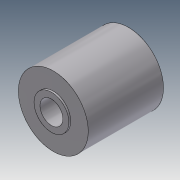
# Autodesk Inventor part: J008110
Saved by Autodesk Inventor 2018.3 (Build 223284000, 284)
## iProperties
Created: 2018-10-11
Material: ALUMINUM, 6061-T651
Vendor: HHMI: JRC - ID&F
Document SubType Name: Modeling
Designer: arnoldj
Density: 2.7 g/cm^3
Appearance: Metal-AL-6061 (Machined)
Part Number: J008110
Description: VP SPACER LOWER CYL
Project: COMMON
RuleStatus: InUse
AfterDocSave0: file://Part Number Cleaner
LAB/DEPT: FLY FACILITY (SHARED RESOURCE)
REQUESTING SCIENTIST: LAVERTY, TODD
SURFACE ROUGHNESS: 64 Ra
DESIGN DEPARTMENT: HHMI: JRC - ID&F
SPECIAL FINISH: NONE
ALTERED ITEM PART NUMBER: N/A
ALTERED ITEM VENDOR: N/A
ALTERED ITEM DESCRIPTION: N/A
Author: arnoldj
Revision Number: -
Autodesk Inventor part; units mm, degrees
ref_plane "YZ Plane" through (0, 0, 0) normal (1, 0, 0) x (0, 1, 0)
ref_plane "XZ Plane" through (0, 0, 0) normal (0, 1, 0) x (-1, 0, 0)
ref_plane "XY Plane" through (0, 0, 0) normal (0, 0, 1) x (1, 0, 0)
sketch "Sketch1" plane through (0, 0, 0) normal (0, 0, 1) x (1, 0, 0)
  line L0 (0, 26.67) -> (0, -26.67) projected
  line L1 (-26.67, 0) -> (26.67, 0) projected
  circle A0 centre (0, 0) radius 19.05
  circle A1 centre (0, 0) radius 6.25
  dimension "d0" = 12.5
  dimension "d1" = 38.1
  constraints: 2 centre point, 2 coincident
  measures "d0" diameter of A1
  measures "d1" diameter of A0
extrude "Extrusion1" add sketch "Sketch1" along normal blind 42.0624 contours A0 L1 A1 L0 | L0 A1 L1 A0 | A0 L0 A1 L1 | L1 A1 L0 A0
sketch "Sketch2" plane through (0, 0, 42.0624) normal (0, 0, 1) x (1, 0, 0)
  circle A0 centre (0, 0) radius 6.25 projected
  circle A1 centre (0, 0) radius 19.05 projected
  circle A2 centre (0, 0) radius 9.5
  dimension "d4" = 19
  constraints: 1 centre point, 1 coincident
  measures "d4" diameter of A2
extrude "Extrusion2" cut sketch "Sketch2" against normal blind 1.016 contours A1
body "Solid1"
